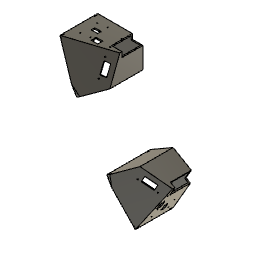
the_case v4.1 (Autodesk Fusion 360 design; units mm, degrees)
Autodesk Fusion 360 part; units mm, degrees
note: some values were not read from the file. Chosen so that the rebuilt part matches the saved one: a direction; where a step ends.
ref_plane "WorkPlane2" through (0, 0, 0) normal (0, 0, 1) x (1, 0, 0) in component "Base"
sketch "top" plane through (0, 0, 0) normal (0, 0, 1) x (1, 0, 0) in component "Base"
  line L0 (-48.3808, 27.2591) -> (41.6192, 27.2591)
  line L1 (41.6192, 27.2591) -> (41.6192, -29.7409)
  line L2 (41.6192, -29.7409) -> (-48.3808, -29.7409)
  line L3 (-48.3808, -29.7409) -> (-48.3808, 27.2591)
  dimension "d1" = 90
  dimension "d2" = 57
  constraint horizontal L0
  constraint vertical L1
  constraint horizontal L2
  constraint vertical L3
  measures "d1" distance of L0.start L0.end
  measures "d2" distance of L0.start L2.end
ref_plane "WorkPlane1" through (-48.3808, -1.2409, 0) normal (-0.866025, 0, -0.5) x (0, 1, 0) in component "Base"
ref_plane "WorkPlane3" through (0, 0, -1) normal (0, 0, 1) x (1, 0, 0) in component "Base"
sketch "start-dot" plane through (0, 0, -1) normal (0, 0, 1) x (1, 0, 0) in component "Base"
  line L0 (-48.3808, -29.7409) -> (-48.3808, 27.2591)
  line L1 (41.6192, -29.7409) -> (-48.3808, -29.7409)
  line L2 (5.6192, -30.7409) -> (-4.3808, -30.7409)
  line L3 (-4.3808, -30.7409) -> (5.6192, -30.7409)
  line L4 (5.6192, -30.7409) -> (15.1298, -27.6507)
  line L5 (5.6192, -30.7409) -> (13, -30.7409) construction
  point P0 (5.6192, -30.7409)
  dimension "d25" = 54
  dimension "d32" = 10
  dimension "d33" = 10
  dimension "d117" = 18
  constraint coincident P0 L2.start
  constraint horizontal L2
  constraint parallel L3 L5
  measures "d25" distance of P0 L0
  measures "d32" distance of P0 L4.end
  measures "d33" distance of P0 L2.end
  measures "d117" angle of L4 L5
ref_plane "WorkPlane3" through (10.3745, -29.1958, -1) normal (0.290381, -0.893701, 0.34202) x (0.951057, 0.309017, 0) in component "Base"
sketch "table-cut" plane through (-48.3808, -1.2409, 0) normal (-0.866025, 0, -0.5) x (0, 1, 0) in component "Base"
  line L0 (-250, -250) -> (250, -250)
  line L1 (250, -250) -> (250, 250)
  line L2 (250, 250) -> (-250, 250)
  line L3 (-250, 250) -> (-250, -250)
  line L4 (-250, -250) -> (250, 250) construction
  line L5 (-250, 250) -> (250, -250) construction
  dimension "d39" = 500
  dimension "d40" = 500
  constraint horizontal L0
  constraint vertical L1
  constraint horizontal L2
  constraint vertical L3
  constraint midpoint origin L5
  measures "d39" distance of L0.start L0.end
  measures "d40" distance of L0.start L2.end
sketch "left-cut" plane through (0, 0, 0) normal (0, 0, 1) x (1, 0, 0) in component "Base"
  line L0 (-250, 250) -> (250, 250)
  line L1 (250, 250) -> (250, -250)
  line L2 (250, -250) -> (-250, -250)
  line L3 (-250, -250) -> (-250, 250)
  line L4 (250, -250) -> (-250, 250) construction
  line L5 (250, 250) -> (-250, -250) construction
  dimension "d41" = 500
  dimension "d42" = 500
  constraint horizontal L0
  constraint vertical L1
  constraint horizontal L2
  constraint vertical L3
  constraint midpoint L4 origin
  measures "d41" distance of L1 L3
  measures "d42" distance of L0.start L2.end
ref_plane "WorkPlane5" through (-3.3808, -29.7409, 0) normal (0, 1, 0) x (-1, 0, 0) in component "Base"
ref_plane "WorkPlane6" through (-3.3808, -59.7409, 0) normal (0, 1, 0) x (-1, 0, 0) in component "Base"
sketch "front-cut" plane through (-3.3808, -59.7409, 0) normal (0, 1, 0) x (1, 0, 0) in component "Base"
  line L0 (-250, -250) -> (250, -250)
  line L1 (250, -250) -> (250, 250)
  line L2 (250, 250) -> (-250, 250)
  line L3 (-250, 250) -> (-250, -250)
  line L4 (250, 250) -> (-250, -250) construction
  line L5 (250, -250) -> (-250, 250) construction
  dimension "d45" = 500
  dimension "d46" = 500
  constraint horizontal L0
  constraint vertical L1
  constraint horizontal L2
  constraint vertical L3
  constraint midpoint origin L4
  measures "d45" distance of L0.start L0.end
  measures "d46" distance of L0.start L2.end
extrude "Extrude1" add sketch "front-cut" along normal blind 500 makes body 1 in component "Base"
extrude "Extrude2" cut sketch "left-cut" against normal blind 500 keep common part bodies 1 in component "Base"
extrude "Extrude3" cut sketch "table-cut" against normal blind 500 keep common part bodies 1 in component "Base"
ref_plane "WorkPlane12" through (-3.3808, 27.2591, 0) normal (0, 1, 0) x (-1, 0, 0) in component "Base"
sketch "back-cut" plane through (-3.3808, 27.2591, 0) normal (0, 1, 0) x (1, 0, 0) in component "Base"
  line L0 (-250, -250) -> (250, -250)
  line L1 (250, -250) -> (250, 250)
  line L2 (250, 250) -> (-250, 250)
  line L3 (-250, 250) -> (-250, -250)
  line L4 (250, 250) -> (-250, -250) construction
  line L5 (250, -250) -> (-250, 250) construction
  dimension "d54" = 500
  dimension "d55" = 500
  constraint horizontal L0
  constraint vertical L1
  constraint horizontal L2
  constraint vertical L3
  constraint midpoint origin L5
  measures "d54" distance of L0.start L0.end
  measures "d55" distance of L0.start L2.end
extrude "Extrude4" cut sketch "back-cut" against normal blind 500 keep common part bodies 1 in component "Base"
ref_plane "WorkPlane10" through (-48.3808, -1.2409, 0) normal (-0.5, 0, 0.866025) x (0, 1, 0) in component "Base"
ref_plane "WorkPlane11" through (-3.3808, -1.2409, -77.9423) normal (-0.5, 0, 0.866025) x (0, 1, 0) in component "Base"
sketch "thumb-cut" plane through (10.3745, -29.1958, -1) normal (0.290381, -0.893701, 0.34202) x (0.939011, 0.334936, 0.077953) in component "Base"
  line L0 (250, -250) -> (-250, -250)
  line L1 (-250, -250) -> (-250, 250)
  line L2 (-250, 250) -> (250, 250)
  line L3 (250, 250) -> (250, -250)
  line L4 (250, -250) -> (-250, 250) construction
  line L5 (-250, -250) -> (250, 250) construction
  dimension "d124" = 500
  dimension "d125" = 500
  dimension "d126" = 500
  constraint horizontal L0
  constraint perpendicular L0 L1
  constraint parallel L0 L2
  constraint parallel L1 L3
  constraint coincident L4 origin
  constraint coincident L5 origin
  measures "d124" distance of L0.start L2.end
  measures "d125" distance of L0.end L1.end
  measures "d126" distance of L1.end L2.end
extrude "Extrude9" cut sketch "thumb-cut" against normal blind 500 keep common part bodies 1 in component "Base"
sketch "Sketch14" plane through (-3.3808, -1.2409, -77.9423) normal (-0.5, 0, 0.866025) x (0, 1, 0) in component "Base"
  line L0 (-250, 250) -> (250, 250)
  line L1 (250, 250) -> (250, -250)
  line L2 (250, -250) -> (-250, -250)
  line L3 (-250, -250) -> (-250, 250)
  line L4 (-250, 250) -> (250, -250) construction
  line L5 (250, 250) -> (-250, -250) construction
  dimension "d129" = 500
  dimension "d130" = 500
  constraint horizontal L0
  constraint perpendicular L0 L1
  constraint parallel L0 L2
  constraint parallel L1 L3
  constraint coincident L4 origin
  constraint coincident L5 origin
  measures "d129" distance of L1.end L2.end
  measures "d130" distance of L0.end L1.end
extrude "Extrude10" cut sketch "Sketch14" along normal blind 500 keep common part bodies 1 in component "Base"
sketch "thumb" plane through (10.3745, -29.1958, -1) normal (0.290381, -0.893701, 0.34202) x (0.939011, 0.334936, 0.077953) in component "Base"
  line L0 (-4.9828, 0.4148) -> (-15.5863, -49.4707)
  line L1 (-15.5863, -49.4707) -> (19.6271, -56.9556)
  line L2 (19.6271, -56.9556) -> (30.2305, -7.07)
  line L3 (30.2305, -7.07) -> (-4.9828, 0.4148)
  line L4 (0, 0) -> (64, 0) construction
  point P0 (-4.9828, 0.4148)
  dimension "d134" = 36
  dimension "d135" = 51
  dimension "d137" = 12
  constraint perpendicular L0 L1
  constraint parallel L0 L2
  constraint parallel L1 L3
  constraint coincident P0 L0.start
  constraint coincident L4.start origin
  constraint horizontal L4
  measures "d134" distance of P0 L2.end
  measures "d135" distance of P0 L0.end
  measures "d137" angle of L3 L4
ref_plane "WorkPlane13" through (39.6804, -30.4029, -29.0352) normal (0.939586, 0.313756, -0.136874) x (0.015035, 0.361638, 0.932197) in component "Base"
sketch "Sketch16" plane through (39.6804, -30.4029, -29.0352) normal (0.939586, 0.313756, -0.136874) x (0.015035, 0.361638, 0.932197) in component "Base"
  line L0 (-250, 250) -> (250, 250)
  line L1 (250, 250) -> (250, -250)
  line L2 (250, -250) -> (-250, -250)
  line L3 (-250, -250) -> (-250, 250)
  line L4 (-250, 250) -> (250, -250) construction
  line L5 (250, 250) -> (-250, -250) construction
  dimension "d163" = 500
  dimension "d164" = 500
  constraint horizontal L0
  constraint perpendicular L0 L1
  constraint parallel L0 L2
  constraint parallel L1 L3
  constraint coincident L4 origin
  constraint coincident L5 origin
  measures "d163" distance of L0.start L0.end
  measures "d164" distance of L0.end L1.end
extrude "Extrude14" [suppressed] in component "Base"
ref_plane "WorkPlane14" through (41.6192, -1.2409, 0) normal (-1, 0, 0) x (0, -1, 0) in component "Base"
sketch "Sketch17" plane through (41.6192, -1.2409, 0) normal (-1, 0, 0) x (0, 1, 0) in component "Base"
  line L0 (250, 250) -> (-250, 250)
  line L1 (-250, 250) -> (-250, -250)
  line L2 (-250, -250) -> (250, -250)
  line L3 (250, -250) -> (250, 250)
  line L4 (250, 250) -> (-250, -250) construction
  line L5 (-250, 250) -> (250, -250) construction
  dimension "d168" = 500
  dimension "d169" = 500
  constraint horizontal L0
  constraint perpendicular L0 L1
  constraint parallel L0 L2
  constraint parallel L1 L3
  constraint coincident L4 origin
  constraint coincident L5 origin
  measures "d168" distance of L1.end L2.end
  measures "d169" distance of L0.end L1.end
extrude "Extrude15" cut sketch "Sketch17" along normal blind 500 keep common part bodies 1 in component "Base"
shell "Shell1" thickness 2.5 removed faces 1 at (-21.705, -1.7409, -46.2038) on bodies 1 in component "Base"
sketch "left_case" plane through (0, 0, 0) normal (0, 0, 1) x (1, 0, 0) in component "left"
  arc A0 (12.49, 2.5) -> (11, 1.01) centre (12.49, 1.01) ccw
  line L0 (14.5, 32) -> (14.5, 25)
  circle A1 centre (27, 45.5) radius 1.1
  arc A2 (47, 61.01) -> (45.51, 62.5) centre (45.51, 61.01) ccw
  line L1 (45.5, 7) -> (45.5, 17)
  arc A3 (23.51, 59.5) -> (25, 60.99) centre (23.51, 60.99) ccw
  line L2 (62, 56.5) -> (62, 18)
  line L3 (32.5, 17) -> (32.5, 7)
  line L4 (62, 18) -> (83, 18)
  line L5 (47, 57.99) -> (47, 61.01)
  arc A4 (81.51, 2.5) -> (83, 3.99) centre (81.51, 3.99) ccw
  arc A5 (-7, -7.01) -> (-5.51, -8.5) centre (-5.51, -7.01) ccw
  arc A6 (26.49, 62.5) -> (25, 61.01) centre (26.49, 61.01) ccw
  line L6 (27.5, 32) -> (14.5, 32)
  line L7 (14.5, 25) -> (27.5, 25)
  line L8 (45.5, 17) -> (32.5, 17)
  circle A7 centre (27, 11.5) radius 1.1
  line L9 (32.5, 7) -> (45.5, 7)
  arc A8 (47, 57.99) -> (48.49, 56.5) centre (48.49, 57.99) ccw
  line L10 (45.51, 62.5) -> (26.49, 62.5)
  circle A9 centre (9, 42.5) radius 1.1
  circle A10 centre (9, 8.5) radius 1.1
  line L11 (-5.51, 59.5) -> (23.51, 59.5)
  arc A11 (9.51, -8.5) -> (11, -7.01) centre (9.51, -7.01) ccw
  arc A12 (-5.51, 59.5) -> (-7, 58.01) centre (-5.51, 58.01) ccw
  line L12 (12.49, 2.5) -> (81.51, 2.5)
  line L13 (11, -7.01) -> (11, 1.01)
  line L14 (27.5, 25) -> (27.5, 32)
  line L15 (62, 56.5) -> (48.49, 56.5)
  line L16 (-7, -7.01) -> (-7, 58.01)
  line L17 (83, 3.99) -> (83, 18)
  line L18 (-5.51, -8.5) -> (9.51, -8.5)
  line L19 (25, 61.01) -> (25, 60.99)
  circle A13 centre (63, 14) radius 1.1
  circle A14 centre (60.5, 39.5) radius 1.1
  line L20 (62, 18) -> (90.5, 18)
  line L21 (90.5, 18) -> (90.5, 64.5)
  line L22 (90.5, 64.5) -> (62, 64.5)
  line L23 (62, 64.5) -> (62, 18)
  constraint horizontal L20
  constraint vertical L21
  constraint horizontal L22
  constraint vertical L23
extrude "Extrude16" cut sketch "left_case" against normal blind 10 contours L2 L4 L20 L21 L22 L23 sketch seen with x (1, 0, 0) y (0, 1, 0) z (0, 0, 1) at (-41.3808, -32.2409, 0) bodies 1 in component "Base"
extrude "Extrude17" cut sketch "left_case" against normal blind 5 contours L0 L6 L7 L14 | A1 | L1 L3 L8 L9 | A7 | A9 | A10 | A13 | A14 sketch seen with x (1, 0, 0) y (0, 1, 0) z (0, 0, 1) at (-41.3808, -32.2409, 0) bodies 1 in component "Base"
sketch "left_pcb_edgecut" plane through (0, 0, 0) normal (0, 0, 1) x (1, 0, 0) in component "left"
  arc A0 (-5.51, 59.5) -> (-7, 58.01) centre (-5.51, 58.01) ccw
  line L0 (45.51, 62.5) -> (26.49, 62.5)
  line L1 (47, 57.99) -> (47, 61.01)
  line L2 (12.49, 2.5) -> (81.51, 2.5)
  arc A1 (23.51, 59.5) -> (25, 60.99) centre (23.51, 60.99) ccw
  arc A2 (-7, -7.01) -> (-5.51, -8.5) centre (-5.51, -7.01) ccw
  arc A3 (47, 57.99) -> (48.49, 56.5) centre (48.49, 57.99) ccw
  arc A4 (26.49, 62.5) -> (25, 61.01) centre (26.49, 61.01) ccw
  line L3 (25, 61.01) -> (25, 60.99)
  line L4 (-7, -7.01) -> (-7, 58.01)
  line L5 (-5.51, -8.5) -> (9.51, -8.5)
  arc A5 (9.51, -8.5) -> (11, -7.01) centre (9.51, -7.01) ccw
  arc A6 (83, 52.01) -> (81.51, 53.5) centre (81.51, 52.01) ccw
  arc A7 (81.51, 2.5) -> (83, 3.99) centre (81.51, 3.99) ccw
  line L6 (83, 3.99) -> (83, 52.01)
  line L7 (63.51, 56.5) -> (48.49, 56.5)
  arc A8 (65, 55.01) -> (63.51, 56.5) centre (63.51, 55.01) ccw
  line L8 (81.51, 53.5) -> (66.49, 53.5)
  line L9 (65, 54.99) -> (65, 55.01)
  arc A9 (65, 54.99) -> (66.49, 53.5) centre (66.49, 54.99) ccw
  line L10 (11, -7.01) -> (11, 1.01)
  arc A10 (47, 61.01) -> (45.51, 62.5) centre (45.51, 61.01) ccw
  line L11 (-5.51, 59.5) -> (23.51, 59.5)
  arc A11 (12.49, 2.5) -> (11, 1.01) centre (12.49, 1.01) ccw
extrude "Extrude3'" add sketch "left_pcb_edgecut" along normal blind 3.6 separate body makes body 2 in component "left"
sketch "thumb_case (1)" plane through (0, 0, 0) normal (0, 0, 1) x (1, 0, 0) in component "thumb"
  arc A0 (27, 41) -> (25.5, 42.5) centre (25.5, 41) ccw
  circle A1 centre (9, 34) radius 1.1
  line L0 (-9, -7) -> (-9, 41)
  arc A2 (25.5, -8.5) -> (27, -7) centre (25.5, -7) ccw
  circle A3 centre (9, 0) radius 1.1
  line L1 (20, 6) -> (20, 28)
  line L2 (-7.5, 42.5) -> (25.5, 42.5)
  line L3 (9, 6) -> (20, 6)
  arc A4 (-9, -7) -> (-7.5, -8.5) centre (-7.5, -7) ccw
  line L4 (9, 28) -> (9, 6)
  arc A5 (-7.5, 42.5) -> (-9, 41) centre (-7.5, 41) ccw
  line L5 (20, 28) -> (9, 28)
  line L6 (-7.5, -8.5) -> (25.5, -8.5)
  line L7 (27, -7) -> (27, 41)
extrude "Extrude3''" add sketch "thumb_case (1)" along normal blind 3.6 separate body contours A0 L0 A2 L2 A4 A5 L6 L7 | L1 L3 L4 L5 makes body 3 in component "thumb"
extrude "Extrude4'" add sketch "thumb_case (1)" along normal blind 11 from surface at 3.6 separate body contours A0 L0 A2 L2 A4 A5 L6 L7 | A1 | A3 | L1 L3 L4 L5 makes body 4 in component "thumb"
extrude "Extrude18" cut sketch "thumb_case (1)" against normal blind 5 contours A1 | A3 | L1 L3 L4 L5 sketch seen with x (0.956793, 0.26555, -0.11845) y (0.015035, 0.361638, 0.932197) z (0.290381, -0.893701, 0.34202) at (13.5914, -43.7205, -41.6844) bodies 1 in component "Base"
extrude "Extrude2'" add sketch "left_pcb_edgecut" along normal blind 11 from surface at 3.6 separate body sketch seen with x (1, 0, 0) y (0, 1, 0) z (0, 0, 1) at (-41.3808, -32.2409, 0) makes body 5
copy_body "CutPasteBodies1" bodies 5 body 5 seen with x (1, 0, 0) y (0, 1, 0) z (0, 0, 1) at (41.3808, 32.2409, 0) removing the originals makes body 6 in component "left"
sketch "Sketch6" plane through (-48.3808, -1.2409, 0) normal (-0.866025, 0, -0.5) x (0, 1, 0)
  circle A0 centre (23, 5.5) radius 4.5
  circle A1 centre (23, 5.5) radius 5.5
  line L0 (-38.01, 0) -> (27.01, 0)
  line L1 (28.5, 0.745) -> (28.5, 15.255)
  circle A2 centre (-42.0143, 5.5) radius 4.5
  circle A3 centre (-42.0143, 5.5) radius 5.5
  line L2 (-46.663, 0) -> (28.5, 0)
  line L3 (-46.663, 0) -> (-58.5, 70.0545)
  circle A4 centre (-53, 84.5) radius 4.5
  circle A5 centre (-53, 84.5) radius 5.5
  circle A6 centre (23, 84.5) radius 4.5
  circle A7 centre (23, 84.5) radius 5.5
  line L4 (-58.5, 90) -> (28.5, 90)
  line L5 (28.5, 90) -> (28.5, 0)
  line L6 (-58.5, 90) -> (-58.5, 70.0545)
  dimension "d210" = 9
  dimension "d211" = 11
  dimension "d212" = 5.5
  dimension "d213" = 5.5
  dimension "d218" = 9
  dimension "d219" = 11
  dimension "d220" = 5.5
  dimension "d221" = 5.5
  dimension "d222" = 9
  dimension "d223" = 11
  dimension "d224" = 9
  dimension "d225" = 11
  dimension "d226" = 5.5
  dimension "d227" = 5.5
  dimension "d228" = 5.5
  dimension "d229" = 5.5
  constraint concentric A0 A1
  constraint concentric A2 A3
  constraint concentric A4 A5
  constraint concentric A6 A7
  measures "d210" diameter of A0
  measures "d211" diameter of A1
  measures "d212" distance of A0.centre L0
  measures "d213" distance of A0.centre L1
  measures "d218" diameter of A2
  measures "d219" diameter of A3
  measures "d220" distance of A2.centre L2
  measures "d221" distance of A2.centre L3
  measures "d222" diameter of A4
  measures "d223" diameter of A5
  measures "d224" diameter of A6
  measures "d225" diameter of A7
  measures "d226" distance of A6.centre L4
  measures "d227" distance of A6.centre L5
  measures "d228" distance of A4.centre L4
  measures "d229" distance of A4.centre L6
extrude "Extrude19" add sketch "Sketch6" along normal up to far side of body 1 contours A0 | A1 | A7 | A3 | A5 | A2 | A4 | A6 bodies 1 in component "Base"
extrude "Extrude20" cut sketch "Sketch6" against normal blind 1 contours A0 | A2 | A4 | A6 bodies 1 in component "Base"
ref_plane "WorkPlane15" through (26.6192, -1.2409, -129.9038) normal (-0.5, 0, 0.866025) x (0, 1, 0) in component "Base"
mirror "Mirror1" about plane through (26.6192, -1.2409, -129.9038) normal (-0.5, 0, 0.866025) of bodies 1 makes body 7 in component "Base"
component "left" placed x (1, 0, 0) y (0, 1, 0) z (0, 0, 1) at (-41.3808, -32.2409, 0)
component "Base" placed x (1, 0, 0) y (0, 1, 0) z (0, 0, 1) at (0, 0, 0)
component "thumb" placed x (0.956793, 0.26555, -0.11845) y (0.015035, 0.361638, 0.932197) z (0.290381, -0.893701, 0.34202) at (13.5914, -43.7205, -41.6844)
equation "angleA = 18 deg"
equation "angleB = 20 deg"
equation "d24 = -dd3"
equation "d25 = dd1"
equation "d26 = dd2"
equation "d31 = 90 deg - angleB"
equation "angleC = 12 deg"
equation "lagre = 50 cm"
equation "d39 = lagre"
equation "d40 = d39"
equation "d41 = lagre"
equation "d42 = d41"
equation "d45 = lagre"
equation "d46 = d45"
equation "d47 = lagre"
equation "d49 = -lagre"
equation "d51 = -lagre"
equation "d54 = lagre"
equation "d55 = lagre"
equation "d56 = -lagre"
equation "dd1 = 54 mm"
equation "dd2 = 1 mm"
equation "dd3 = 1 mm"
equation "pcb_with_hot_swap = 3.6 mm"
equation "d117 = angleA"
equation "d124 = lagre"
equation "d126 = lagre"
equation "d127 = -lagre"
equation "d129 = lagre"
equation "d130 = lagre"
equation "d131 = lagre"
equation "d136 = dd2"
equation "d137 = angleC"
equation "nn_depth_from_pcb = 10 mm"
equation "d163 = lagre"
equation "d164 = lagre"
equation "d165 = -lagre"
equation "d168 = lagre"
equation "d169 = lagre"
equation "d170 = lagre"
equation "d180 = -nn_depth_from_pcb"
equation "d186 = pcb_with_hot_swap"
equation "d188 = pcb_with_hot_swap"
equation "d190 = pcb_with_hot_swap"
equation "d207 = pcb_with_hot_swap"
equation "d212 = ( 11 / 2 ) * 1 mm"
